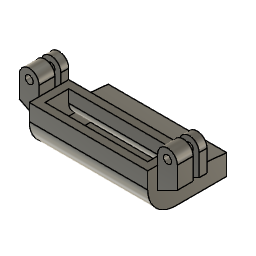
Biqu b2 fan duct (Autodesk Fusion 360 design; units mm, degrees)
Autodesk Fusion 360 part; units mm, degrees
sketch "Sketch1" plane through (0, 0, 0) normal (0, 1, 0) x (1, 0, 0)
  line L0 (-15, -2.5) -> (15, -2.5)
  line L1 (15, -2.5) -> (15, 3.7)
  line L2 (15, 3.7) -> (-15, 3.7)
  line L3 (-15, 3.7) -> (-15, -2.5)
  line L4 (13.5, -1.5) -> (-13.5, -1.5)
  line L5 (-13.5, -1.5) -> (-13.5, 3.1)
  line L6 (-13.5, 3.1) -> (13.5, 3.1)
  line L7 (13.5, 3.1) -> (13.5, -1.5)
  dimension "d1" = 6.2
  dimension "d2" = 30
  dimension "d3" = 15
  dimension "d4" = 2.5
  dimension "d14" = 1
  dimension "d15" = 0.6
  dimension "d16" = 1.5
  dimension "d17" = 1.5
  constraint horizontal L0
  constraint vertical L1
  constraint horizontal L2
  constraint vertical L3
  constraint horizontal L4
  constraint vertical L5
  constraint horizontal L6
  constraint vertical L7
  measures "d1" distance of L0.end L1.end
  measures "d2" distance of L0.start L0.end
  measures "d3" horizontal distance of origin L0.start
  measures "d4" vertical distance of origin L0.end
  measures "d14" distance of L0 L4
  measures "d15" distance of L2 L6
  measures "d16" distance of L1 L7
  measures "d17" distance of L3 L5
extrude "Extrude1" add sketch "Sketch1" along normal blind 10 makes body 1
draft "Draft1" angle 5 neutral plane through (0, 0, 0) pull (0, -1, 0) 1 faces at (4.5, 3.3333, 1.5) on bodies 1
chamfer "Chamfer1" distance 1 distance2 10 1 edges at (0, 10, 2.5) measured on face at (-4.5, 10, 1.875) on bodies 1
sketch "Sketch4" plane through (0, 0, 0) normal (0, -1, 0) x (1, 0, 0)
  line L0 (13.5, -3.1) -> (-13.5, -3.1)
  line L1 (-13.5, -3.1) -> (-13.5, 1.5)
  line L2 (-13.5, 1.5) -> (13.5, 1.5)
  line L3 (13.5, 1.5) -> (13.5, -3.1)
  line L4 (-15, 2.5) -> (-15, -3.7)
  line L5 (-15, -3.7) -> (15, -3.7)
  line L6 (15, -3.7) -> (15, 2.5)
  line L7 (15, 2.5) -> (-15, 2.5)
  line L8 (-15, 2.5) -> (15, 2.5)
  line L9 (15, 2.5) -> (15, -3.7)
  line L10 (15, -3.7) -> (-15, -3.7)
  line L11 (-15, -3.7) -> (-15, 2.5)
  line L12 (13.5, -3.1) -> (-13.5, -3.1)
  line L13 (-13.5, -3.1) -> (-13.5, 1.5)
  line L14 (-13.5, 1.5) -> (13.5, 1.5)
  line L15 (13.5, 1.5) -> (13.5, -3.1)
  constraint horizontal L8
  constraint vertical L9
  constraint horizontal L10
  constraint vertical L11
  constraint coincident L5.end L6.start
  constraint coincident L4.start L7.end
  constraint horizontal L12
  constraint vertical L13
  constraint horizontal L14
  constraint vertical L15
  constraint coincident L1.end L2.start
  constraint coincident L0.start L3.end
extrude "Extrude4" add sketch "Sketch4" along normal blind 8 separate body makes body 2
sketch "Sketch6" plane through (0, -8, 0) normal (0, -1, 0) x (1, 0, 0)
  line L0 (-13.5, 1.5) -> (13.5, 1.5)
  line L1 (13.5, 1.5) -> (13.5, -3.1)
  line L2 (13.5, -3.1) -> (-13.5, -3.1)
  line L3 (-13.5, -3.1) -> (-13.5, 1.5)
  line L4 (-15, -3.7) -> (15, -3.7)
  line L5 (15, -3.7) -> (15, 2.5)
  line L6 (15, 2.5) -> (-15, 2.5)
  line L7 (-15, 2.5) -> (-15, -3.7)
  line L8 (-15, 2.5) -> (15, 2.5)
  line L9 (15, 2.5) -> (15, -3.7)
  line L10 (15, -3.7) -> (-15, -3.7)
  line L11 (-15, -3.7) -> (-15, 2.5)
  constraint horizontal L8
  constraint vertical L9
  constraint horizontal L10
  constraint vertical L11
  constraint coincident L4.end L5.start
  constraint coincident L6.end L7.start
extrude "Extrude6" add sketch "Sketch6" along normal blind 2 contours L0 L1 L2 L3 | L4 L5 L6 L7 L8 L9 L10 L11 bodies 2
sketch "Sketch7" plane through (0, 0, 2.5) normal (0, 0, 1) x (-1, 0, 0)
  line L0 (-15, 0) -> (15, 0)
  line L1 (15, 0) -> (15, 10)
  line L2 (15, 10) -> (-15, 10)
  line L3 (-15, 10) -> (-15, 0)
  line L4 (-15, 10) -> (15, 10)
  line L5 (15, 10) -> (15, 0)
  line L6 (15, 0) -> (-15, 0)
  line L7 (-15, 0) -> (-15, 10)
  line L8 (-13, 8) -> (13, 8)
  line L9 (13, 8) -> (13, 2)
  line L10 (13, 2) -> (-13, 2)
  line L11 (-13, 2) -> (-13, 8)
  dimension "d32" = 2
  dimension "d33" = 2
  dimension "d34" = 2
  dimension "d35" = 2
  constraint horizontal L4
  constraint vertical L5
  constraint horizontal L6
  constraint vertical L7
  constraint coincident L0.end L1.start
  constraint coincident L2.end L3.start
  constraint horizontal L8
  constraint vertical L9
  constraint horizontal L10
  constraint vertical L11
  measures "d32" distance of L4 L8
  measures "d33" distance of L7 L11
  measures "d34" distance of L6 L10
  measures "d35" distance of L5 L9
extrude "Extrude7" cut sketch "Sketch7" against normal blind 4 contours L8 L9 L10 L11 bodies 2
fillet "Fillet1" radius 4 tangency weight 1.43006 1 edges at (0, -8, -3.1) on bodies 2
extrude "Extrude8" add sketch "Sketch7" along normal blind 5 bodies 2 1
fillet "Fillet2" radius 2.5 1 edges at (0, 0, 2.5) on bodies 2
fillet "Fillet3" radius 7 1 edges at (0, -10, -3.7) on bodies 2
sketch "Sketch8" plane through (0, 0, 0) normal (0, 1, 0) x (-1, 0, 0)
  line L0 (-15, 4.7625) -> (15, 4.7625)
  line L1 (15, 4.7625) -> (15, 7.5)
  line L2 (15, 7.5) -> (-15, 7.5)
  line L3 (-15, 7.5) -> (-15, 4.7625)
  line L4 (-15, 10) -> (-15, 4.5)
  line L5 (-20, 4.5) -> (-20, 10)
  circle A0 centre (-17.5, 10) radius 1
  arc A1 (-15, 10) -> (-20, 10) centre (-17.5, 10) ccw
  line L6 (-20, 4.5) -> (-15, 2)
  line L7 (-15, 2) -> (-15, 4.5)
  line L8 (15, 10) -> (15, 4.5)
  arc A2 (15, 10) -> (10, 10) centre (12.5, 10) ccw
  line L9 (15, 2) -> (15, 4.5)
  circle A3 centre (12.5, 10) radius 1
  line L10 (10, 4.5) -> (10, 10)
  line L11 (10, 4.5) -> (15, 2)
  line L12 (15, 7.5) -> (15, 4.7625)
  line L13 (15, -3.7) -> (15, 1.5)
  circle A4 centre (17.5, 10) radius 1
  line L14 (20, 4.5) -> (15, 2)
  line L15 (15, 7.5) -> (15, 4.7625)
  line L16 (15, 4.7625) -> (15, 7.5)
  line L17 (15, 10) -> (15, 4.5)
  line L18 (15, 2) -> (15, 4.5)
  line L19 (20, 4.5) -> (20, 10)
  arc A5 (20, 10) -> (15, 10) centre (17.5, 10) ccw
  dimension "d46" = 5
  dimension "d48" = 3
  dimension "d49" = 2
  dimension "d50" = 2.5
  dimension "d52" = 5.5
  dimension "d53" = 2.5
  dimension "d60" = 5
  dimension "d61" = 3
  dimension "d62" = 2
  dimension "d63" = 2.5
  dimension "d64" = 5.5
  dimension "d65" = 2.5
  constraint vertical L4
  constraint vertical L5
  constraint tangent L4 A1
  constraint tangent L5 A1
  constraint equal L4 L5
  constraint coincident L2.end L4
  constraint vertical L8
  constraint vertical L10
  constraint tangent L8 A2
  constraint tangent A2 L10
  constraint equal L8 L10
  constraint coincident L1.end L8
  constraint symmetric L0.end L13 L1.start
  constraint symmetric L1.end L13 L2.start
  constraint symmetric A2.end L13 L19.end
  constraint symmetric L8.start L13 A2.start
  constraint symmetric L8.end L13 L9.end
  constraint symmetric L10.start L13 L14.start
  constraint symmetric L9.start L13 L11.end
  constraint symmetric A2 L13 A5
  constraint symmetric A3 L13 A4
  measures "d46" distance of L5.end L4.start
  measures "d48" distance of L2.end L4.end
  measures "d49" diameter of A0
  measures "d50" distance of L4 A0.centre
  measures "d52" distance of L5.end L5.start
  measures "d53" distance of L4.start A0.centre
  measures "d60" distance of A2.end L8.start
  measures "d61" distance of L8.end L1.end
  measures "d62" diameter of A3
  measures "d63" distance of A2.centre L8
  measures "d64" distance of A2.end L10.start
  measures "d65" distance of L8.start A2.centre
extrude "Extrude9" add sketch "Sketch8" against normal blind 2 contours L3 L4 L5 A1 L6 L7 bodies 2
extrude "Extrude10" add sketch "Sketch8" against normal blind 4 from surface at -3.5 contours L3 L4 L5 A1 L6 L7 bodies 2
extrude "Extrude11" add sketch "Sketch8" against normal blind 2 contours L1 L8 L9 L12 L14 L15 L16 L17 L18 L19 A5 bodies 2
extrude "Extrude12" add sketch "Sketch8" against normal blind 4 from surface at -3.5 contours L1 L8 L9 L12 L14 L15 L16 L17 L18 L19 A5 bodies 2
fillet "Fillet4" radius 3 1 edges at (0, -2, 1.5) on bodies 2
sketch "Sketch9" plane through (0, 0, -3.7) normal (0, 0, -1) x (1, 0, 0)
  line L0 (15, 3) -> (-15, 3)
  line L1 (-15, 3) -> (-15, -10)
  line L2 (-15, -10) -> (15, -10)
  line L3 (15, -10) -> (15, 3)
  line L4 (13.5, -4) -> (-13.5, -4)
  line L5 (-13.5, -4) -> (-13.5, -10)
  line L6 (-13.5, -10) -> (13.5, -10)
  line L7 (13.5, -10) -> (13.5, -4)
  dimension "d75" = 1.5
  dimension "d76" = 1.5
  dimension "d77" = 6
  constraint horizontal L4
  constraint vertical L5
  constraint horizontal L6
  constraint vertical L7
  constraint coincident L2 L5.end
  measures "d75" distance of L3 L7
  measures "d76" distance of L1 L5
  measures "d77" distance of L4 L6
extrude "Extrude13" cut sketch "Sketch9" against normal blind 2 contours L2 L4 L5 L6 L7 bodies 2
sketch "Sketch11" plane through (-13.5, 0, 0) normal (1, 0, 0) x (0, 1, 0)
  line L0 (10, -3.7) -> (10, 0.6251)
  line L1 (10, 0.6251) -> (0, 1.5)
  line L2 (0, 1.5) -> (-8, 1.5)
  line L3 (-8, 1.5) -> (-8, 0.9)
  spline S0 degree 3 poles (-8, 0.9) (-8, 0.2684) (-7.9268, -0.3912) (-7.5637, -1.372) (-7.36, -1.7261) (-6.8247, -2.3037) (-6.524, -2.5177) (-5.875, -2.8289) (-5.5417, -2.9295) (-4.809, -3.0705) (-4.4008, -3.1) (-4, -3.1) knots 0 0 0 0 0.189491 0.189491 0.313115 0.313115 0.425243 0.425243 0.528589 0.528589 0.648678 0.648678 0.648678 0.648678
  line L4 (-4, -3.1) -> (4, -3.1)
  line L5 (4, -3.1) -> (4, -3.7)
  line L6 (4, -3.7) -> (10, -3.7)
  line L7 (10, 0.6251) -> (10, -1.5)
  line L8 (10, -1.5) -> (9, -1.5)
  line L9 (9, -1.5) -> (5, 1.0626)
  line L10 (5, 1.0626) -> (10, 0.6251)
  line L11 (10, 0.6251) -> (10, -1.5)
  constraint coincident L0.end L1.start
  constraint coincident L0 L7.end
  constraint perpendicular L7 L8
  constraint midpoint L1 L9.end
extrude "Extrude15" add sketch "Sketch11" along normal up to surface (27 mm away) contours L0 L1 L7 L8 L9 L10 L11 bodies 2
